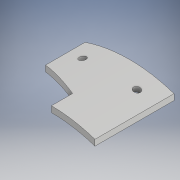
# Autodesk Inventor part: cap_mount
Saved by Autodesk Inventor 2019 (Build 230136000, 136)
## iProperties
Created: 2019-01-26
Part Number: cap_mount
Material: Generic
Document SubType Name: Modeling
Designer: Brian
Density: 1 g/cm^3
Appearance: Default
Author: Brian
Autodesk Inventor part; units mm, degrees
ref_plane "YZ Plane" through (0, 0, 0) normal (1, 0, 0) x (0, 1, 0)
sketch "Sketch1" plane through (0, 0, 0) normal (0, 1, 0) x (-1, 0, 0)
  line L0 (0, 0) -> (0, -45) construction
  arc A0 (0, -45) -> (0, 0) centre (-66.2854, -22.5) ccw
  line L1 (0, 0) -> (3, 0)
  line L2 (0, -45) -> (3, -45)
  arc A1 (3, -45) -> (3, 0) centre (-63.2854, -22.5) ccw
  dimension "d0" = 45
  dimension "d1" = 70
  dimension "d2" = 3
  dimension "d3" = 3
  dimension "d4" = 70
  constraints: 6 end point, 4 point on circle, 2 centre point, 2 horizontal, 1 vertical
  measures "d0" distance of L0.start L0.end
  measures "d1" radius of A0
  measures "d2" distance of L0.start L1.end
  measures "d3" distance of L0.end L2.end
  measures "d4" radius of A1
extrude "Extrusion1" add sketch "Sketch1" along normal blind 40
ref_plane "Work Plane1" through (-3, 0, -45) normal (-0.9469, 0, -0.3214) x (0, -1, 0)
sketch "Sketch2" plane through (-3, 0, -45) normal (-0.9469, 0, -0.3214) x (0, -1, 0)
  line L0 (-40, 42.612) -> (-40, 0) projected
  line L1 (0, -0.9643) -> (-40, -0.9643) projected
  point P0 (0, 41.6477)
  point P1 (-30, 9.0357)
  dimension "d7" = 10
  dimension "d8" = 10
  measures "d7" distance from line of L0 point (-30, 9.036)
  measures "d8" distance from line of L1 point (-30, 9.036)
hole "Hole1" at (-5.9043, 30, -36.4438) direction (0.9469, 0, 0.3214) diameter 3.5 end through all
ref_plane "Work Plane2" through (-3, 0, 0) normal (-0.9469, 0, 0.3214) x (0, -1, 0)
sketch "Sketch3" plane through (-3, 0, 0) normal (-0.9469, 0, 0.3214) x (0, -1, 0)
  line L0 (0, 0.9643) -> (-40, 0.9643) projected
  line L1 (-40, 0) -> (-40, -42.612) projected
  point P0 (-30, -9.0357)
  dimension "d16" = 10
  dimension "d17" = 10
  measures "d16" distance from line of L0 point (-30, -9.036)
  measures "d17" distance from line of L1 point (-30, -9.036)
hole "Hole2" at (-5.9043, 30, -8.5562) direction (0.9469, 0, -0.3214) diameter 3.5 end through all
sketch "Sketch4" plane through (0, 0, 0) normal (1, 0, 0) x (0, 1, 0)
  line L0 (0, -45) -> (40, -45) projected
  line L1 (0, 0) -> (40, 0) projected
  line L2 (0, -45) -> (0, 0) projected
  line L3 (0, 0) -> (40, 0) projected
  line L4 (40, -45) -> (40, 0) projected
  line L5 (0, -45) -> (40, -45) projected
  line L6 (0, 0) -> (0, -22)
  line L7 (20, -45) -> (10.7074, -22)
  line L8 (10.7074, -22) -> (0, -22)
  line L9 (20, -45) -> (0, -45)
  line L10 (0, -22) -> (0, -45)
  point P0 (30, -7.0213)
  point P1 (30, -34.518)
  point P2 (20, 0)
  dimension "d25" = 22
  dimension "d26" = 112
  constraints: 10 end point, 2 midpoint, 1 collinear, 1 horizontal, 1 perpendicular, 1 point on line, 2 other
  measures "d25" distance of L2.end L6.end
  measures "d26" angle of L0 L7
extrude "Extrusion2" cut sketch "Sketch4" against normal up to next contours L2 L8 L7 L0
body "Solid1"
